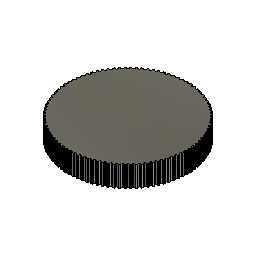
gear_92z (Autodesk Fusion 360 design; units mm, degrees)
Autodesk Fusion 360 part; units mm, degrees
sketch "Sketch1" plane through (0, 0, 0) normal (0, 0, 1) x (1, 0, 0) in component "gt2 pulley"
  circle A0 centre (0, 0) radius 29.2845 construction
  circle A1 centre (0, 0) radius 28.2805 construction
  line L0 (0, 0) -> (0, 29.2845) construction
  line L1 (0, 0) -> (0.9998, 29.2674) construction
  line L2 (0, 0) -> (1.4043, 29.2508) construction
  circle A2 centre (0, 0) radius 29.0305 construction
  arc A3 (0.3974, 28.8948) -> (0.476, 28.5962) centre (1.3921, 28.9971) ccw
  circle A4 centre (0, 0) radius 28.8805 construction
  arc A5 (0.2494, 29.0294) -> (0, 29.0305) centre (0, 0) ccw
  arc A6 (0.3974, 28.8948) -> (0.2494, 29.0294) centre (0.2482, 28.8794) ccw
  arc A7 (0.476, 28.5962) -> (0.9655, 28.264) centre (0.9845, 28.8187) ccw
  arc A8 (0, 29.0305) -> (-0.2494, 29.0294) centre (0, 0) ccw
  arc A9 (-0.2494, 29.0294) -> (-0.3974, 28.8948) centre (-0.2482, 28.8794) ccw
  arc A10 (-0.476, 28.5962) -> (-0.3974, 28.8948) centre (-1.3921, 28.9971) ccw
  arc A11 (-0.9657, 28.264) -> (-0.476, 28.5962) centre (-0.9845, 28.8187) ccw
  arc A12 (0.9655, 28.264) -> (-0.9655, 28.264) centre (0, 0) ccw
  point P0 (1.3921, 28.9971)
  point P1 (0, 29.0305)
  dimension "d18" = 58.569
  dimension "d19" = 1.957
  dimension "d22" = 1.004
  dimension "d24" = 0.75
  dimension "d26" = 1
  dimension "d27" = 0.15
  dimension "d28" = 0.15
  dimension "d47" = 0.555
  dimension "d52" = 3.812
  constraint coincident A0.centre A1.centre
  constraint coincident A0 L0.end
  constraint vertical L0
  constraint coincident A0 L1.end
  constraint coincident A0 L2.end
  constraint concentric A1 A2
  constraint coincident A1 A7.end
  constraint coincident L1 A7.end
  constraint coincident A2 P0
  constraint coincident L2 P0
  constraint coincident P0 A3.centre
  constraint coincident A2 P1
  constraint coincident L0 P1
  constraint concentric A2 A4
  constraint coincident P1 A5.end
  constraint coincident A4 A6.centre
  constraint coincident A3.start A6.start
  constraint tangent A3 A6
  constraint tangent A3 A7
  constraint symmetric L0 A7.end A12.end
  constraint symmetric L0 A3.start A9.end
  constraint symmetric L0 A3.end A10.start
  constraint symmetric L0 A3 A10
  constraint symmetric L0 A5.start A8.end
  constraint symmetric L0 P1 A5.end
  constraint symmetric L0 A5 A8
  constraint symmetric L0 A6 A9
  constraint symmetric L0 A7 A11
  constraint coincident A1 A11.start
  constraint tangent A1 A7
  constraint coincident L1 A7.centre
  measures "d18" diameter of A0
  measures "d19" angle of L0 L1
  measures "d22" distance of A0 A1
  measures "d24" distance of A1 A2
  measures "d26" radius of A3
  measures "d27" distance of A2 A4
  measures "d28" radius of A6
  measures "d47" radius of A7
extrude "Extrude1" add sketch "Sketch1" along normal blind 10 makes body 1
pattern_circular "C-Pattern1" count 92 over 360 about axis through (0, 0, 1.75) along (0, 0, 1) of bodies 1 makes body 2 at (-2.037, 28.207, 6.6667) makes body 3 at (-3.1055, 28.1095, 3.3333) makes body 4 at (-6.2782, 27.5748, 6.6667) makes body 5 at (-7.5267, 27.2605, 6.6667) makes body 6 at (-8.7596, 26.8897, 3.3333) makes body 7 at (-11.952, 25.6308, 6.6667) makes body 8 at (-12.3395, 25.4465, 3.3333) makes body 9 at (-14.7857, 24.1074, 6.6667) makes body 10 at (-16.3964, 23.0422, 6.6667) makes body 11 at (-17.2586, 22.4037, 3.3333) makes body 12 at (-19.3813, 20.595, 6.6667) makes body 13 at (-20.7416, 19.2243, 6.6667) makes body 14 at (-22.4038, 17.2585, 6.6667) makes body 15 at (-22.6631, 16.9166, 3.3333) makes body 16 at (-23.7647, 15.3306, 3.3333) makes body 17 at (-24.7555, 13.6731, 3.3333) makes body 18 at (-26.2293, 10.574, 6.6667) makes body 19 at (-26.8898, 8.7594, 6.6667) makes body 20 at (-27.4248, 6.904, 6.6667) makes body 21 at (-27.7106, 5.6487, 6.6667) makes body 22 at (-27.905, 4.5935, 6.6667) makes body 23 at (-28.1534, 2.6785, 3.3333) makes body 24 at (-28.2803, -0.1074, 6.6667) makes body 25 at (-28.207, -2.037, 6.6667) makes body 26 at (-28.0023, -3.9572, 6.6667) makes body 27 at (-27.667, -5.8589, 6.6667) makes body 28 at (-27.4248, -6.9041, 3.3333) makes body 29 at (-26.8897, -8.7596, 3.3333) makes body 30 at (-25.6308, -11.952, 6.6667) makes body 31 at (-25.4465, -12.3395, 3.3333) makes body 32 at (-24.5451, -14.0472, 3.3333) makes body 33 at (-23.0422, -16.3964, 6.6667) makes body 34 at (-21.8696, -17.9307, 6.6667) makes body 35 at (-20.595, -19.3813, 6.6667) makes body 36 at (-19.2243, -20.7416, 6.6667) makes body 37 at (-17.2585, -22.4038, 6.6667) makes body 38 at (-16.9166, -22.6631, 3.3333) makes body 39 at (-14.7856, -24.1075, 6.6667) makes body 40 at (-13.6731, -24.7555, 3.3333) makes body 41 at (-10.574, -26.2293, 6.6667) makes body 42 at (-8.7594, -26.8898, 6.6667) makes body 43 at (-7.5265, -27.2606, 6.6667) makes body 44 at (-5.6487, -27.7106, 6.6667) makes body 45 at (-4.5935, -27.905, 3.3333) makes body 46 at (-2.6785, -28.1534, 3.3333) makes body 47 at (0.1074, -28.2803, 6.6667) makes body 48 at (2.037, -28.207, 6.6667) makes body 49 at (3.9572, -28.0023, 6.6667) makes body 50 at (5.0165, -27.832, 3.3333) makes body 51 at (6.9041, -27.4248, 3.3333) makes body 52 at (8.7596, -26.8897, 3.3333) makes body 53 at (11.952, -25.6308, 6.6667) makes body 54 at (13.1061, -25.0603, 6.6667) makes body 55 at (14.0472, -24.5451, 3.3333) makes body 56 at (16.3964, -23.0422, 6.6667) makes body 57 at (17.2586, -22.4037, 3.3333) makes body 58 at (19.8451, -20.1484, 6.6667) makes body 59 at (20.1485, -19.845, 3.3333) makes body 60 at (22.4038, -17.2585, 6.6667) makes body 61 at (22.6631, -16.9166, 3.3333) makes body 62 at (23.7647, -15.3306, 3.3333) makes body 63 at (24.7555, -13.6731, 3.3333) makes body 64 at (25.9818, -11.1684, 6.6667) makes body 65 at (26.6834, -9.3693, 6.6667) makes body 66 at (27.4248, -6.904, 6.6667) makes body 67 at (27.5264, -6.4871, 3.3333) makes body 68 at (28.0315, -3.7445, 6.6667) makes body 69 at (28.1534, -2.6785, 3.3333) makes body 70 at (28.2803, 0.1074, 6.6667) makes body 71 at (28.207, 2.037, 6.6667) makes body 72 at (28.0023, 3.9572, 6.6667) makes body 73 at (27.832, 5.0165, 3.3333) makes body 74 at (27.4248, 6.9041, 3.3333) makes body 75 at (26.8897, 8.7596, 3.3333) makes body 76 at (25.6308, 11.952, 6.6667) makes body 77 at (25.0603, 13.1061, 6.6667) makes body 78 at (24.5451, 14.0472, 3.3333) makes body 79 at (23.0422, 16.3964, 6.6667) makes body 80 at (22.4037, 17.2586, 3.3333) makes body 81 at (20.1484, 19.8451, 6.6667) makes body 82 at (19.845, 20.1485, 3.3333) makes body 83 at (17.2585, 22.4038, 6.6667) makes body 84 at (16.9166, 22.6631, 3.3333) makes body 85 at (15.3306, 23.7647, 6.6667) makes body 86 at (13.6731, 24.7555, 3.3333) makes body 87 at (10.574, 26.2293, 6.6667) makes body 88 at (9.3693, 26.6834, 6.6667) makes body 89 at (7.5265, 27.2606, 6.6667) makes body 90 at (6.4871, 27.5264, 3.3333) makes body 91 at (3.7445, 28.0315, 6.6667) makes body 92 at (1.8228, 28.2217, 6.6667)
sketch "Sketch2" plane through (0, 0, 10) normal (0, 0, 1) x (-1, 0, 0)
  arc A0 (-8.1784, -27.7161) -> (-8.0722, -27.8857) centre (-8.0306, -27.7416) ccw
  arc A1 (-8.0722, -27.8857) -> (-7.5919, -28.0202) centre (0, 0) ccw
  arc A2 (-7.5919, -28.0202) -> (-7.4131, -27.9305) centre (-7.5526, -27.8755) ccw
  arc A3 (-7.2568, -27.6642) -> (-7.4131, -27.9305) centre (-6.4828, -28.2974) ccw
  arc A4 (-6.6958, -27.4764) -> (-7.2568, -27.6642) centre (-6.8272, -28.0156) ccw
  arc A5 (-8.5553, -26.9554) -> (-6.6958, -27.4764) centre (0, 0) ccw
  arc A6 (-8.1735, -27.4073) -> (-8.5553, -26.9554) centre (-8.7232, -27.4844) ccw
  arc A7 (-8.1784, -27.7161) -> (-8.1735, -27.4073) centre (-9.1638, -27.5462) ccw
  circle A8 centre (0, 0) radius 28.2805
  constraint concentric A1 A8
extrude "Extrude2" add sketch "Sketch2" against normal blind 10 contours A5 A8 bodies 1 2 3 4 5 6 7 8 9 10 11 12 13 14 15 16 17 18 19 20 21 22 23 24 25 26 27 28 29 30 31 32 33 34 35 36 37 38 39 40 41 42 43 44 45 46 47 48 49 50 51 52 53 54 55 56 57 58 59 60 61 62 63 64 65 66 67 68 69 70 71 72 73 74 75 76 77 78 79 80 81 82 83 84 85 86 87 88 89 90 91 92
extrude "Extrude4" [suppressed] in component "gt2 pulley"
pattern_circular "C-Pattern7" [suppressed] in component "gt2 pulley"
extrude "Extrude3" [suppressed] in component "gt2 pulley"
pattern_circular "C-Pattern6" [suppressed] in component "gt2 pulley"
extrude "Extrude2'" [suppressed] in component "gt2 pulley"
pattern_circular "C-Pattern5" [suppressed] in component "gt2 pulley"
extrude "Extrude1'" [suppressed] in component "gt2 pulley"
pattern_circular "C-Pattern4" [suppressed] in component "gt2 pulley"
pattern_circular "C-Pattern3" [suppressed] in component "gt2 pulley"
pattern_circular "C-Pattern2" [suppressed] in component "gt2 pulley"
pattern_circular "C-Pattern1'" [suppressed] in component "gt2 pulley"
copy_body "Body->Comp1" [suppressed] in component "Component"
copy_body "Body->Comp2" [suppressed] in component "Component'"
copy_body "Body->Comp3" [suppressed] in component "Component''"
copy_body "Body->Comp4" [suppressed] in component "Component'''"
copy_body "Body->Comp5" [suppressed] in component "Component''''"
copy_body "Body->Comp6" [suppressed] in component "Component'''''"
copy_body "Body->Comp7" [suppressed] in component "Component''''''"
copy_body "Body->Comp8" [suppressed] in component "Component'''''''"
copy_body "Body->Comp9" [suppressed] in component "Component''''''''"
copy_body "Body->Comp10" [suppressed] in component "Component'''''''''"
copy_body "Body->Comp11" [suppressed] in component "Component''''''''''"
copy_body "Body->Comp12" [suppressed] in component "Component'''''''''''"
copy_body "Body->Comp13" [suppressed] in component "Component''''''''''''"
copy_body "Body->Comp14" [suppressed] in component "Component'''''''''''''"
copy_body "Body->Comp15" [suppressed] in component "Component''''''''''''''"
copy_body "Body->Comp16" [suppressed] in component "Component'''''''''''''''"
copy_body "Body->Comp17" [suppressed] in component "Component''''''''''''''''"
copy_body "Body->Comp18" [suppressed] in component "Component'''''''''''''''''"
copy_body "Body->Comp19" [suppressed] in component "Component''''''''''''''''''"
copy_body "Body->Comp20" [suppressed] in component "Component'''''''''''''''''''"
component "gt2 pulley" placed x (1, 0, 0) y (0, 1, 0) z (0, 0, 1) at (0, 0, 0)
equation "NumTeeth = 92" comment "min 20"
equation "ToothPitch = 2 mm"
equation "PullyDia = NumTeeth * ToothPitch / PI"
equation "ToothAng = ( ( 360 / NumTeeth ) * 1 deg )"
equation "TransOffsetAngle = ToothAng * 0.2"
equation "Sholulder_Radius = 0.15 mm"
equation "Root_Radius = 0.555 mm"
equation "TransRadius = 1 mm"
equation "ToolHeight = 0.75 mm"
equation "PLD = 0.254 mm"
equation "d18 = PullyDia"
equation "d19 = ToothAng / 2"
equation "d22 = PLD + ToolHeight"
equation "d24 = ToolHeight"
equation "d26 = TransRadius"
equation "d27 = Sholulder_Radius"
equation "d31 = NumTeeth"
equation "d33 = NumTeeth"
equation "d35 = NumTeeth"
equation "d37 = NumTeeth"
equation "d41 = NumTeeth"
equation "d45 = NumTeeth"
equation "d47 = Root_Radius"
equation "d50 = NumTeeth"
